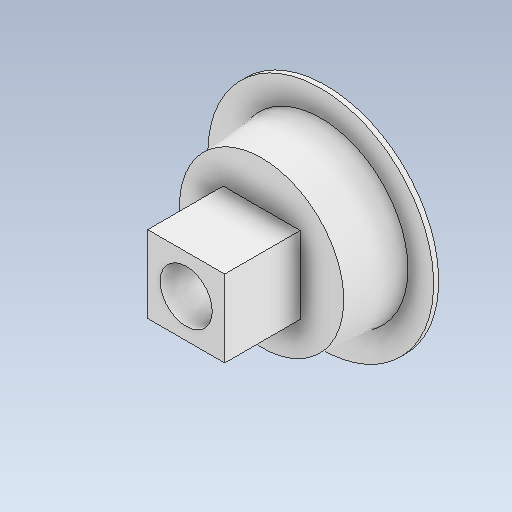
# Autodesk Inventor part: Seil_Rolle_Antrieb_Links
Saved by Autodesk Inventor 2021 (Build 250183000, 183)
## iProperties
Created: 2022-06-29
Part Number: Seil_Rolle_Antrieb_Links
Material: PC/ABS-Kunststoff
Document SubType Name: Modeling
Designer: adria
Mass: 4.38282 g
Surface Area: 58.4928 cm^2
Volume: 12.2674 cm^3
Density: 0.357273 g/cm^3
Appearance: Glatt - Weiß
Author: adria
Autodesk Inventor part; units mm, degrees
ref_plane "YZ Plane" through (0, 0, 0) normal (1, 0, 0) x (0, 1, 0)
ref_plane "XZ Plane" through (0, 0, 0) normal (0, 1, 0) x (-1, 0, 0)
ref_plane "XY Plane" through (0, 0, 0) normal (0, 0, 1) x (1, 0, 0)
sketch "Skizze1" plane through (0, 0, 0) normal (0, 1, 0) x (-1, 0, 0)
  line L0 (17, 1) -> (22, 1)
  line L1 (22, 1) -> (22, 0)
  line L2 (22, 0) -> (0, 0)
  line L3 (0, 12.5) -> (0, 0)
  line L4 (99.15, 0) -> (-16.525, 0) projected
  line L5 (0, -2.5) -> (0, 15) projected
  line L6 (16, 12.5) -> (0, 12.5)
  arc A0 (16, 12.5) -> (17, 1) centre (82.625, 12.5) ccw
  line L7 (16, 12.5) -> (16, 0) construction
  dimension "d5" = 44
  dimension "d6" = 12.5
  dimension "d7" = 1
  dimension "d15" = 16
  dimension "d16" = 17
  constraints: 13 end point, 3 horizontal, 2 point on circle, 1 centre point, 1 perpendicular, 1 point on line, 1 tangent, 1 vertical
  measures "d5" diameter of L1 L5
  measures "d6" distance of L2.end L3.start
  measures "d7" distance of L0.end L1.end
  measures "d15" distance of L6.start L3.start
  measures "d16" distance from line of L3 L0.start
revolve "Umdrehung1" add sketch "Skizze1" angle 360 about axis through (0, 0, 12.5) along (0, 0, -1)
sketch "Skizze3" plane through (0, 0, 12.5) normal (0, 0, 1) x (1, 0, 0)
  circle A0 centre (0, 0) radius 22 projected
  circle A1 centre (0, 0) radius 5.075
  dimension "d8" = 10.15
  constraints: 1 centre point, 1 coincident
  measures "d8" diameter of A1
extrude "Extrusion2" cut sketch "Skizze3" against normal through all contours A1
sketch "Skizze4" plane through (0, 0, 12.5) normal (0, 0, 1) x (1, 0, 0)
  circle A0 centre (0, 0) radius 5.075 projected
  circle A1 centre (0, 0) radius 16 projected
  line L0 (-7.5, -7.5) -> (7.5, -7.5)
  line L1 (7.5, -7.5) -> (7.5, 7.5)
  line L2 (7.5, 7.5) -> (-7.5, 7.5)
  line L3 (-7.5, 7.5) -> (-7.5, -7.5)
  line L4 (-7.5, -7.5) -> (7.5, 7.5) construction
  line L5 (7.5, -7.5) -> (-7.5, 7.5) construction
  dimension "d11" = 15
  dimension "d12" = 15
  constraints: 12 end point, 2 midpoint, 2 parallel, 1 horizontal, 1 perpendicular
  measures "d11" distance of L2.end L1.end
  measures "d12" distance of L1.end L0.end
extrude "Extrusion3" add sketch "Skizze4" along normal blind 14.7 contours L3 L2 L1 L0
